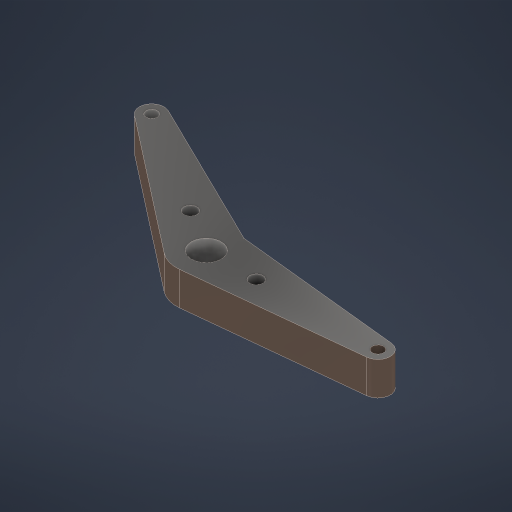
# Autodesk Inventor part: Lever
Saved by Autodesk Inventor 2023 (Build 270158000, 158)
## iProperties
Created: 2022-11-28
Part Number: Lever
Material: Steel
Document SubType Name: Modeling
Designer: iusti
Density: 7.85 g/cm^3
Appearance: Gunmetal - Antique Polished
Author: iusti
Autodesk Inventor part; units mm, degrees
ref_plane "YZ Plane" through (0, 0, 0) normal (1, 0, 0) x (0, 1, 0)
ref_plane "XZ Plane" through (0, 0, 0) normal (0, 1, 0) x (-1, 0, 0)
ref_plane "XY Plane" through (0, 0, 0) normal (0, 0, 1) x (1, 0, 0)
sketch "Sketch1" plane through (0, 0, 0) normal (0, 1, 0) x (-1, 0, 0)
  arc A0 (-0.9262, 8.9522) -> (5.5294, 7.1011) centre (0, 0) ccw construction
  arc A1 (42.0471, -30.6137) -> (45.9477, -24.3715) centre (43.6745, -27.2908) ccw
  arc A2 (-51.8808, 3.6804) -> (-51.8808, -3.6804) centre (-51.5, 0) ccw
  line L0 (0, 0) -> (-51.5, 0) construction
  line L1 (0, 0) -> (43.6745, -27.2908) construction
  line L2 (-0.9262, 8.9522) -> (-51.8808, 3.6804)
  line L3 (-51.8808, -3.6804) -> (-2.5197, -8.7873)
  line L4 (-3.9585, -8.0827) -> (-2.5197, -8.7873) construction
  line L5 (45.9477, -24.3715) -> (5.5294, 7.1011)
  line L6 (-2.5197, -8.7873) -> (42.0471, -30.6137)
  line L7 (-2.5197, -8.7873) -> (-0.9262, -8.9522) construction
  arc A3 (5.5294, 7.1011) -> (-0.9262, 8.9522) centre (0, 0) ccw
  circle A4 centre (-15, 0) radius 2
  circle A5 centre (12.7207, -7.9488) radius 2
  circle A6 centre (43.6745, -27.2908) radius 1.7
  circle A7 centre (-51.5, 0) radius 1.7
  circle A8 centre (0, 0) radius 4.5
  dimension "d6" = 18
  dimension "d7" = 7.4
  dimension "d8" = 7.4
  dimension "d9" = 32
  dimension "d10" = 51.5
  dimension "d11" = 51.5
  dimension "d14" = 4
  dimension "d15" = 4
  dimension "d16" = 3.4
  dimension "d17" = 3.4
  dimension "d18" = 15
  dimension "d19" = 15
  dimension "d20" = 9
  constraints: 16 end point, 12 tangent, 10 point on circle, 9 centre point, 4 coincident, 2 point on line, 1 horizontal, 1 horizontal alignment
  measures "d6" diameter of A0
  measures "d7" diameter of A1
  measures "d8" diameter of A2
  measures "d9" angle of L1 L0
  measures "d10" distance of L0.start L1.end
  measures "d11" distance of L0.start L0.end
  measures "d14" diameter of A4
  measures "d15" diameter of A5
  measures "d16" diameter of A6
  measures "d17" diameter of A7
  measures "d18" distance of point (0, 0) A5.centre
  measures "d19" distance of point (0, 0) A4.centre
  measures "d20" diameter of A8
extrude "Extrusion1" add sketch "Sketch1" along normal blind 10
body "Solid1"
